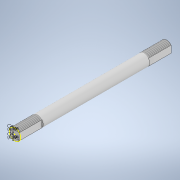
# Autodesk Inventor part: Rear Axle2
Saved by Autodesk Inventor 2021 (Build 250183000, 183)
## iProperties
Created: 2021-02-13
Part Number: Rear Axle2
Material: Generic
Document SubType Name: Modeling
Designer: bl17
Density: 1 g/cm^3
Appearance: Default
Author: bl17
Autodesk Inventor part; units mm, degrees
ref_plane "YZ Plane" through (0, 0, 0) normal (1, 0, 0) x (0, 1, 0)
ref_plane "XZ Plane" through (0, 0, 0) normal (0, 1, 0) x (-1, 0, 0)
ref_plane "XY Plane" through (0, 0, 0) normal (0, 0, 1) x (1, 0, 0)
sketch "Sketch1" plane through (0, 0, 0) normal (0, 0, 1) x (1, 0, 0)
  circle A0 centre (0, 0) radius 6.35
  dimension "d0" = 12.7
  constraints: 1 centre point, 1 coincident
  measures "d0" diameter of A0
extrude "Extrusion1" add sketch "Sketch1" along normal blind 170
sketch "Sketch2" plane through (0, 0, 170) normal (0, 0, 1) x (1, 0, 0)
  circle A0 centre (0, 0) radius 6.35 projected
  line L0 (-5, 3.9144) -> (5, 3.9144) construction
  line L1 (-5, 3.9144) -> (5, 3.9144) construction
  line L2 (-5, -3.9144) -> (5, -3.9144) construction
  line L3 (-5, -3.9144) -> (5, -3.9144) construction
  circle A1 centre (0, 0) radius 6.35 projected
  dimension "d3" = 10
  dimension "d4" = 0
  dimension "d5" = 10
  dimension "d6" = 0
  constraints: 8 end point, 4 horizontal, 4 point on circle, 2 collinear
  measures "d3" distance of L0.start L0.end
  measures "d4" distance between parallel lines of L0 L1
  measures "d5" distance of L2.start L2.end
  measures "d6" distance between parallel lines of L2 L3
thread "Thread1" size "1/2-13 UNC" class "2A" standard "ANSI Unified Screw Threads" length 25.4
thread "Thread2" size "1/2-13 UNC" class "2A" standard "ANSI Unified Screw Threads" length 25.4
sketch "Sketch3" plane through (0, 0, 170) normal (0, 0, 1) x (1, 0, 0)
  circle A0 centre (0, 0) radius 6.35 projected
  line L0 (5.0019, 3.912) -> (5.0019, -3.912)
  arc A1 (5.0019, -3.912) -> (5.0019, 3.912) centre (0, 0) ccw
  constraints: 5 point on circle, 2 end point, 1 centre point, 1 coincident, 1 concentric, 1 vertical
extrude "Extrusion2" cut sketch "Sketch3" against normal blind 25.4 contours A0 L0 picked at (5.2474, -0.9063)
sketch "Sketch4" plane through (0, 0, 170) normal (0, 0, 1) x (1, 0, 0)
  arc A0 (5.0019, 3.912) -> (5.0019, -3.912) centre (0, 0) ccw projected
  line L0 (-5.0019, 3.912) -> (-5.0019, -3.912)
  arc A1 (-5.0019, 3.912) -> (-5.0019, -3.912) centre (0, 0) ccw
  constraints: 4 point on circle, 2 end point, 1 centre point, 1 coincident, 1 vertical
extrude "Extrusion3" cut sketch "Sketch4" against normal blind 25.4
sketch "Sketch5" plane through (0, 0, 0) normal (0, 0, -1) x (-1, 0, 0)
  line L0 (-5.0019, -3.912) -> (-5.0019, 3.912) projected
  line L1 (-5.0019, 3.912) -> (-5.0019, -3.912)
  arc A0 (-5.0019, 3.912) -> (-5.0019, -3.912) centre (0, 0) ccw
  constraints: 2 end point, 2 point on circle, 1 centre point, 1 coincident, 1 collinear
extrude "Extrusion4" cut sketch "Sketch5" against normal blind 25.4
sketch "Sketch6" plane through (0, 0, 0) normal (0, 0, -1) x (-1, 0, 0)
  arc A0 (5.0019, -3.912) -> (5.0019, 3.912) centre (0, 0) ccw projected
  line L0 (5.0019, 3.912) -> (5.0019, -3.912)
  arc A1 (5.0019, -3.912) -> (5.0019, 3.912) centre (0, 0) ccw
  constraints: 2 end point, 2 point on circle, 1 centre point, 1 coincident, 1 vertical
extrude "Extrusion5" cut sketch "Sketch6" against normal blind 25.4
body "Solid1"
